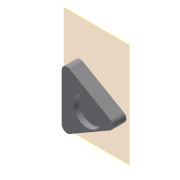
# Autodesk Inventor part: cellSTORM_v5_beamaligner
Saved by Autodesk Inventor 2019.4 (Build 234330000, 330)
## iProperties
Created: 2020-06-28
Part Number: cellSTORM_v5_beamaligner
Material: Generic
Document SubType Name: Modeling
Designer: diederichbenedict
Density: 1 g/cm^3
Appearance: Default
Author: diederichbenedict
Autodesk Inventor part; units mm, degrees
ref_plane "YZ Plane" through (0, 0, 0) normal (1, 0, 0) x (0, 1, 0)
ref_plane "XZ Plane" through (0, 0, 0) normal (0, 1, 0) x (-1, 0, 0)
ref_plane "XY Plane" through (0, 0, 0) normal (0, 0, 1) x (1, 0, 0)
ref_plane "Work Plane1" through (0, 0, 0) normal (0, 0, 1) x (1, 0, 0)
sketch "Sketch1" plane through (0, 0, 0) normal (0, 0, 1) x (1, 0, 0)
  arc A0 (2.9803, -1.8351) -> (2.9803, 1.8351) centre (0, 0) ccw construction
  line L0 (-4.0197, 6.5098) -> (-4.0197, 18.8449) construction
  line L1 (-12.9369, 22.9677) -> (-4.0197, 18.8449) construction
  line L2 (-18.8679, 22.9677) -> (-12.9369, 22.9677) construction
  line L3 (-18.8679, 22.9677) -> (-18.8679, -12.7323) construction
  line L4 (-18.8679, -12.7323) -> (-4.0197, -12.7323) construction
  line L5 (-4.0197, -12.7323) -> (-4.0197, -6.5098) construction
  line L6 (3.6372, -2.0891) -> (-4.0197, -6.5098) construction
  line L7 (3.6372, 2.0891) -> (3.6372, -2.0891) construction
  line L8 (-4.0197, 6.5098) -> (3.6372, 2.0891) construction
  circle A1 centre (-13, 7.5056) radius 1.4 construction
  circle A2 centre (-13, -7.5056) radius 1.4 construction
  circle A3 centre (0, 0) radius 1.4 construction
  ellipse E0 centre (13.6585, -10.0323) end of major axis (13.6585, -11.0323) minor radius 0.7071 construction
  ellipse E1 centre (18.2547, 10.4677) end of major axis (18.2547, 9.4677) minor radius 0.7071 construction
  ellipse E2 centre (33.4575, -5.0323) end of major axis (33.4575, -6.0323) minor radius 0.7071 construction
  line L9 (-4.0197, 6.5098) -> (4.2556, 1.7321) construction
  arc A4 (4.2556, -1.7321) -> (4.2556, 1.7321) centre (3.2556, 0) ccw construction
  line L10 (4.2556, -1.7321) -> (-4.0197, -6.5098) construction
  line L11 (-4.0197, -12.7323) -> (-4.0197, -6.5098) construction
  line L12 (38.7608, -12.7323) -> (-4.0197, -12.7323) construction
  line L13 (38.7608, 18.8449) -> (38.7608, -12.7323) construction
  line L14 (38.7608, 18.8449) -> (31.9614, 18.8449) construction
  line L15 (31.9614, 3.9677) -> (31.9614, 18.8449) construction
  line L16 (31.9614, 3.9677) -> (32.2848, 3.9677) construction
  line L17 (32.2848, 3.9677) -> (32.2848, -7.9947) construction
  line L18 (32.2848, -7.9947) -> (16.4885, -7.9947) construction
  line L19 (16.4885, -7.9947) -> (16.4885, 3.9677) construction
  line L20 (16.4885, 3.9677) -> (19.2761, 3.9677) construction
  line L21 (19.2761, 18.8449) -> (19.2761, 3.9677) construction
  line L22 (-4.0197, 18.8449) -> (19.2761, 18.8449) construction
  line L23 (-4.0197, 6.5098) -> (-4.0197, 18.8449) construction
  circle A5 centre (-6.1405, -0.0323) radius 5 construction
  line L24 (0, 0) -> (-13, -7.5056)
  line L25 (-13, -7.5056) -> (-13, 7.5056) construction
  line L26 (-13, 7.5056) -> (0, 0) construction
  line L27 (2.5664, -1.7321) -> (-12.7832, -10.5941)
  line L28 (-15.7832, -8.8621) -> (-15.7832, 8.8621)
  line L29 (-12.7832, 10.5941) -> (2.5664, 1.7321)
  arc A6 (-12.7832, 10.5941) -> (-15.7832, 8.8621) centre (-13.7832, 8.8621) ccw
  arc A7 (-15.7832, -8.8621) -> (-12.7832, -10.5941) centre (-13.7832, -8.8621) ccw
  arc A8 (2.5664, -1.7321) -> (2.5664, 1.7321) centre (1.5664, 0) ccw
  circle A9 centre (-13, 7.5056) radius 1.95
  circle A10 centre (0, 0) radius 1.95
  circle A11 centre (-13, -7.5056) radius 1.95
  point P0 (0, 0)
  point P1 (-8.6667, 0)
  dimension "d0" = 2
  dimension "d1" = 3.9
  dimension "d2" = 3.9
  dimension "d3" = 3.9
  constraints: 12 end point, 6 centre point, 6 point on circle, 6 tangent, 4 coincident, 2 equal radius, 12 other
  measures "d0" radius of A6
  measures "d1" diameter of A9
  measures "d2" diameter of A10
  measures "d3" diameter of A11
extrude "Extrusion1" add sketch "Sketch1" along normal blind 3
sketch "Sketch2" plane through (0, 0, 3) normal (0, 0, 1) x (1, 0, 0)
  circle A0 centre (-13, -7.5056) radius 1.95 projected
  circle A1 centre (0, 0) radius 1.95 projected
  circle A2 centre (-13, 7.5056) radius 1.95 projected
  line L0 (-15.7832, 8.8621) -> (-15.7832, -8.8621) projected
  arc A3 (-15.7832, -8.8621) -> (-12.7832, -10.5941) centre (-13.7832, -8.8621) ccw projected
  line L1 (-12.7832, -10.5941) -> (2.5664, -1.7321) projected
  arc A4 (2.5664, -1.7321) -> (2.5664, 1.7321) centre (1.5664, 0) ccw projected
  line L2 (2.5664, 1.7321) -> (-12.7832, 10.5941) projected
  arc A5 (-12.7832, 10.5941) -> (-15.7832, 8.8621) centre (-13.7832, 8.8621) ccw projected
  point P0 (0, 0)
extrude "Extrusion2" add sketch "Sketch2" along normal blind 2 contours A0 | A1 | A2 | A5 L2 A4 L1 A3 L0
sketch "Sketch3" plane through (0, 0, 5) normal (0, 0, 1) x (1, 0, 0)
  circle A0 centre (-6.1405, -0.0323) radius 5 projected
  circle A1 centre (-6.1405, -0.0323) radius 5.25
  point P0 (0, 0)
  dimension "d8" = 0.25
  constraints: 1 centre point
  measures "d8" radial gap between concentric circles of A0 A1
extrude "Extrusion3" cut sketch "Sketch3" against normal blind 1.9 contours A0 | A1
body "Solid1"
